Autodesk Fusion 360 part; units mm, degrees
(part 5 of 18)
  spline S23 degree 5 poles (23.1879, -24.3163) (23.1865, -24.3123) (23.1838, -24.3044) (23.1798, -24.2926) (23.1744, -24.2768) (23.1676, -24.2571) (23.1608, -24.2375) (23.154, -24.2179) (23.1471, -24.1984) (23.1403, -24.1789) (23.1334, -24.1595) (23.1265, -24.1401) (23.1197, -24.1208) (23.1128, -24.1016) (23.1058, -24.0823) (23.0989, -24.0632) (23.092, -24.0441) (23.085, -24.025) (23.078, -24.006) (23.071, -23.9871) (23.064, -23.9681) (23.057, -23.9493) (23.05, -23.9305) (23.0429, -23.9118) (23.0359, -23.8931) (23.0288, -23.8744) (23.0217, -23.8558) (23.0147, -23.8373) (23.0076, -23.8188) (23.0004, -23.8004) (22.9933, -23.782) (22.9862, -23.7637) (22.979, -23.7454) (22.9719, -23.7272) (22.9647, -23.7091) (22.9575, -23.691) (22.9503, -23.6729) (22.9431, -23.6549) (22.9359, -23.637) (22.9287, -23.6191) (22.9215, -23.6012) (22.9142, -23.5835) (22.907, -23.5658) (22.8997, -23.5481) (22.8924, -23.5305) (22.8851, -23.5129) (22.8778, -23.4954) (22.8705, -23.478) (22.8632, -23.4606) (22.8559, -23.4433) (22.8486, -23.426) (22.8413, -23.4088) (22.8339, -23.3916) (22.8266, -23.3745) (22.8192, -23.3575) (22.8119, -23.3405) (22.8045, -23.3236) (22.7971, -23.3067) (22.7897, -23.2899) (22.7823, -23.2731) (22.7749, -23.2564) (22.7675, -23.2398) (22.7601, -23.2232) (22.7527, -23.2067) (22.7453, -23.1902) (22.7379, -23.1738) (22.7304, -23.1575) (22.723, -23.1412) (22.7156, -23.125) (22.7081, -23.1088) (22.7007, -23.0927) (22.6932, -23.0766) (22.6858, -23.0607) (22.6783, -23.0447) (22.6709, -23.0289) (22.6634, -23.0131) (22.6559, -22.9973) (22.6485, -22.9816) (22.641, -22.966) (22.6335, -22.9505) (22.626, -22.935) (22.6186, -22.9195) (22.6111, -22.9042) (22.6036, -22.8888) (22.5961, -22.8736) (22.5886, -22.8584) (22.5811, -22.8433) (22.5737, -22.8282) (22.5662, -22.8132) (22.5587, -22.7983) (22.5512, -22.7834) (22.5437, -22.7686) (22.5363, -22.7539) (22.5288, -22.7392) (22.5213, -22.7246) (22.5138, -22.71) (22.5064, -22.6955) (22.4989, -22.6811) (22.4914, -22.6668) (22.484, -22.6525) (22.4765, -22.6383) (22.469, -22.6241) (22.4616, -22.61) (22.4541, -22.596) (22.4467, -22.582) (22.4392, -22.5681) (22.4318, -22.5543) (22.4244, -22.5406) (22.417, -22.5269) (22.4095, -22.5132) (22.4021, -22.4997) (22.3947, -22.4862) (22.3873, -22.4728) (22.3799, -22.4594) (22.3725, -22.4462) (22.3652, -22.4329) (22.3578, -22.4198) (22.3504, -22.4067) (22.3431, -22.3937) (22.3358, -22.3808) (22.3284, -22.3679) (22.3211, -22.3551) (22.3138, -22.3424) (22.3065, -22.3298) (22.2992, -22.3172) (22.2919, -22.3047) (22.2847, -22.2922) (22.2774, -22.2799) (22.2702, -22.2676) (22.2629, -22.2554) (22.2557, -22.2432) (22.2485, -22.2312) (22.2413, -22.2192) (22.2342, -22.2072) (22.227, -22.1954) (22.2199, -22.1836) (22.2127, -22.1719) (22.2056, -22.1603) (22.1985, -22.1487) (22.1915, -22.1372) (22.1844, -22.1258) (22.1774, -22.1145) (22.1703, -22.1033) (22.1633, -22.0921) (22.1564, -22.081) (22.1494, -22.07) (22.1424, -22.059) (22.1355, -22.0482) (22.1286, -22.0374) (22.1217, -22.0267) (22.1149, -22.0161) (22.108, -22.0055) (22.1012, -21.995) (22.0944, -21.9847) (22.0877, -21.9743) (22.0809, -21.9641) (22.0742, -21.954) (22.0675, -21.9439) (22.0609, -21.9339) (22.0542, -21.924) (22.0476, -21.9142) (22.041, -21.9045) (22.0345, -21.8948) (22.028, -21.8853) (22.0215, -21.8758) (22.015, -21.8664) (22.0086, -21.8571) (22.0022, -21.8478) (21.9958, -21.8387) (21.9895, -21.8296) (21.9832, -21.8207) (21.9769, -21.8118) (21.9707, -21.803) (21.9645, -21.7943) (21.9583, -21.7857) (21.9522, -21.7771) (21.9461, -21.7687) (21.9401, -21.7603) (21.9341, -21.7521) (21.9281, -21.7439) (21.9222, -21.7358) (21.9163, -21.7279) (21.9105, -21.72) (21.9047, -21.7122) (21.899, -21.7045) (21.8933, -21.6969) (21.8876, -21.6893) (21.882, -21.6819) (21.8764, -21.6746) (21.8709, -21.6674) (21.8654, -21.6602) (21.86, -21.6532) (21.8547, -21.6463) (21.8494, -21.6394) (21.8441, -21.6327) (21.8389, -21.6261) (21.8338, -21.6195) (21.8287, -21.6131) (21.8237, -21.6068) (21.8187, -21.6005) (21.8138, -21.5944) (21.8089, -21.5884) (21.8042, -21.5825) (21.7994, -21.5767) (21.7948, -21.571) (21.7902, -21.5654) (21.7857, -21.5599) (21.7812, -21.5546) (21.7769, -21.5493) (21.7726, -21.5442) (21.7683, -21.5391) (21.7642, -21.5342) (21.7601, -21.5294) (21.7561, -21.5247) (21.7522, -21.5201) (21.7484, -21.5157) (21.7446, -21.5114) (21.741, -21.5071) (21.7374, -21.5031) (21.7339, -21.4991) (21.7305, -21.4952) (21.7273, -21.4915) (21.7241, -21.4879) (21.721, -21.4845) (21.718, -21.4811) (21.7151, -21.4779) (21.7123, -21.4749) (21.7096, -21.4719) (21.707, -21.4691) (21.7046, -21.4665) (21.7022, -21.464) (21.7, -21.4616) (21.6979, -21.4593) (21.696, -21.4573) (21.6941, -21.4553) (21.6924, -21.4535) (21.6909, -21.4519) (21.6894, -21.4504) (21.6881, -21.4491) (21.687, -21.4479) (21.686, -21.4469) (21.6854, -21.4462) (21.685, -21.4458) (21.6847, -21.4456) (21.6846, -21.4454) knots -1 -1 -1 -1 -1 -1 -0.99583333 -0.99166667 -0.9875 -0.98333333 -0.97916667 -0.975 -0.97083333 -0.96666667 -0.9625 -0.95833333 -0.95416667 -0.95 -0.94583333 -0.94166667 -0.9375 -0.93333333 -0.92916667 -0.925 -0.92083333 -0.91666667 -0.9125 -0.90833333 -0.90416667 -0.9 -0.89583333 -0.89166667 -0.8875 -0.88333333 -0.87916667 -0.875 -0.87083333 -0.86666667 -0.8625 -0.85833333 -0.85416667 -0.85 -0.84583333 -0.84166667 -0.8375 -0.83333333 -0.82916667 -0.825 -0.82083333 -0.81666667 -0.8125 -0.80833333 -0.80416667 -0.8 -0.79583333 -0.79166667 -0.7875 -0.78333333 -0.77916667 -0.775 -0.77083333 -0.76666667 -0.7625 -0.75833333 -0.75416667 -0.75 -0.74583333 -0.74166667 -0.7375 -0.73333333 -0.72916667 -0.725 -0.72083333 -0.71666667 -0.7125 -0.70833333 -0.70416667 -0.7 -0.69583333 -0.69166667 -0.6875 -0.68333333 -0.67916667 -0.675 -0.67083333 -0.66666667 -0.6625 -0.65833333 -0.65416667 -0.65 -0.64583333 -0.64166667 -0.6375 -0.63333333 -0.62916667 -0.625 -0.62083333 -0.61666667 -0.6125 -0.60833333 -0.60416667 -0.6 -0.59583333 -0.59166667 -0.5875 -0.58333333 -0.57916667 -0.575 -0.57083333 -0.56666667 -0.5625 -0.55833333 -0.55416667 -0.55 -0.54583333 -0.54166667 -0.5375 -0.53333333 -0.52916667 -0.525 -0.52083333 -0.51666667 -0.5125 -0.50833333 -0.50416667 -0.5 -0.49583333 -0.49166667 -0.4875 -0.48333333 -0.47916667 -0.475 -0.47083333 -0.46666667 -0.4625 -0.45833333 -0.45416667 -0.45 -0.44583333 -0.44166667 -0.4375 -0.43333333 -0.42916667 -0.425 -0.42083333 -0.41666667 -0.4125 -0.40833333 -0.40416667 -0.4 -0.39583333 -0.39166667 -0.3875 -0.38333333 -0.37916667 -0.375 -0.37083333 -0.36666667 -0.3625 -0.35833333 -0.35416667 -0.35 -0.34583333 -0.34166667 -0.3375 -0.33333333 -0.32916667 -0.325 -0.32083333 -0.31666667 -0.3125 -0.30833333 -0.30416667 -0.3 -0.29583333 -0.29166667 -0.2875 -0.28333333 -0.27916667 -0.275 -0.27083333 -0.26666667 -0.2625 -0.25833333 -0.25416667 -0.25 -0.24583333 -0.24166667 -0.2375 -0.23333333 -0.22916667 -0.225 -0.22083333 -0.21666667 -0.2125 -0.20833333 -0.20416667 -0.2 -0.19583333 -0.19166667 -0.1875 -0.18333333 -0.17916667 -0.175 -0.17083333 -0.16666667 -0.1625 -0.15833333 -0.15416667 -0.15 -0.14583333 -0.14166667 -0.1375 -0.13333333 -0.12916667 -0.125 -0.12083333 -0.11666667 -0.1125 -0.10833333 -0.10416667 -0.1 -0.09583333 -0.09166667 -0.0875 -0.08333333 -0.07916667 -0.075 -0.07083333 -0.06666667 -0.0625 -0.05833333 -0.05416667 -0.05 -0.04583333 -0.04166667 -0.0375 -0.03333333 -0.02916667 -0.025 -0.02083333 -0.01666667 -0.0125 -0.00833333 -0.00416667 0 0 0 0 0 0
  line L46 (21.6846, -21.4454) -> (21.6836, -21.4445)
  line L47 (21.6836, -21.4445) -> (20.5306, -20.3042)
  arc A24 (20.5306, -20.3042) -> (22.339, -18.2958) centre (0, 0) ccw
  line L48 (22.339, -18.2958) -> (23.5936, -19.3233)
  line L49 (23.5936, -19.3233) -> (23.5946, -19.3241)
  spline S24 degree 5 poles (23.5946, -19.3241) (23.5948, -19.3242) (23.595, -19.3245) (23.5955, -19.3248) (23.5962, -19.3254) (23.5973, -19.3263) (23.5986, -19.3273) (23.6001, -19.3284) (23.6017, -19.3297) (23.6035, -19.3311) (23.6054, -19.3326) (23.6076, -19.3342) (23.6098, -19.336) (23.6123, -19.3378) (23.6149, -19.3398) (23.6176, -19.3418) (23.6205, -19.344) (23.6236, -19.3462) (23.6268, -19.3486) (23.6301, -19.3511) (23.6336, -19.3536) (23.6372, -19.3562) (23.641, -19.3589) (23.6449, -19.3618) (23.649, -19.3646) (23.6531, -19.3676) (23.6574, -19.3707) (23.6619, -19.3738) (23.6665, -19.377) (23.6712, -19.3802) (23.676, -19.3836) (23.6809, -19.387) (23.686, -19.3905) (23.6912, -19.394) (23.6965, -19.3976) (23.702, -19.4013) (23.7076, -19.4051) (23.7132, -19.4089) (23.7191, -19.4127) (23.725, -19.4166) (23.731, -19.4206) (23.7372, -19.4246) (23.7434, -19.4287) (23.7498, -19.4329) (23.7563, -19.4371) (23.7629, -19.4413) (23.7696, -19.4456) (23.7764, -19.4499) (23.7834, -19.4543) (23.7904, -19.4587) (23.7975, -19.4632) (23.8048, -19.4677) (23.8121, -19.4723) (23.8196, -19.4769) (23.8271, -19.4816) (23.8348, -19.4862) (23.8426, -19.491) (23.8504, -19.4957) (23.8584, -19.5005) (23.8665, -19.5054) (23.8746, -19.5103) (23.8829, -19.5152) (23.8913, -19.5201) (23.8997, -19.5251) (23.9083, -19.5301) (23.9169, -19.5352) (23.9257, -19.5402) (23.9345, -19.5453) (23.9434, -19.5505) (23.9525, -19.5556) (23.9616, -19.5608) (23.9708, -19.5661) (23.9801, -19.5713) (23.9895, -19.5766) (23.999, -19.5819) (24.0086, -19.5872) (24.0182, -19.5926) (24.028, -19.5979) (24.0379, -19.6033) (24.0478, -19.6088) (24.0578, -19.6142) (24.0679, -19.6197) (24.0781, -19.6252) (24.0884, -19.6307) (24.0988, -19.6362) (24.1092, -19.6417) (24.1198, -19.6473) (24.1304, -19.6529) (24.1411, -19.6585) (24.1519, -19.6641) (24.1628, -19.6697) (24.1737, -19.6754) (24.1848, -19.6811) (24.1959, -19.6867) (24.2071, -19.6924) (24.2184, -19.6981) (24.2297, -19.7039) (24.2412, -19.7096) (24.2527, -19.7154) (24.2643, -19.7211) (24.276, -19.7269) (24.2878, -19.7327) (24.2996, -19.7385) (24.3115, -19.7443) (24.3235, -19.7501) (24.3356, -19.7559) (24.3478, -19.7618) (24.36, -19.7676) (24.3723, -19.7735) (24.3847, -19.7793) (24.3971, -19.7852) (24.4097, -19.7911) (24.4223, -19.797) (24.435, -19.8029) (24.4477, -19.8088) (24.4606, -19.8147) (24.4735, -19.8206) (24.4865, -19.8265) (24.4995, -19.8324) (24.5126, -19.8383) (24.5258, -19.8443) (24.5391, -19.8502) (24.5525, -19.8561) (24.5659, -19.8621) (24.5794, -19.868) (24.5929, -19.874) (24.6065, -19.8799) (24.6202, -19.8859) (24.634, -19.8918) (24.6479, -19.8978) (24.6618, -19.9037) (24.6757, -19.9097) (24.6898, -19.9156) (24.7039, -19.9216) (24.7181, -19.9275) (24.7324, -19.9335) (24.7467, -19.9395) (24.7611, -19.9454) (24.7755, -19.9514) (24.7901, -19.9573) (24.8046, -19.9633) (24.8193, -19.9692) (24.834, -19.9751) (24.8488, -19.9811) (24.8637, -19.987) (24.8786, -19.993) (24.8936, -19.9989) (24.9087, -20.0048) (24.9238, -20.0107) (24.939, -20.0166) (24.9542, -20.0226) (24.9695, -20.0285) (24.9849, -20.0344) (25.0004, -20.0403) (25.0159, -20.0462) (25.0314, -20.052) (25.0471, -20.0579) (25.0628, -20.0638) (25.0785, -20.0697) (25.0943, -20.0755) (25.1102, -20.0814) (25.1262, -20.0872) (25.1422, -20.0931) (25.1583, -20.0989) (25.1744, -20.1047) (25.1906, -20.1105) (25.2068, -20.1164) (25.2232, -20.1222) (25.2395, -20.1279) (25.256, -20.1337) (25.2725, -20.1395) (25.289, -20.1453) (25.3056, -20.151) (25.3223, -20.1568) (25.3391, -20.1625) (25.3559, -20.1682) (25.3727, -20.1739) (25.3896, -20.1796) (25.4066, -20.1853) (25.4236, -20.191) (25.4407, -20.1967) (25.4579, -20.2023) (25.4751, -20.208) (25.4923, -20.2136) (25.5097, -20.2192) (25.527, -20.2248) (25.5445, -20.2304) (25.562, -20.236) (25.5795, -20.2416) (25.5971, -20.2471) (25.6148, -20.2527) (25.6325, -20.2582) (25.6503, -20.2637) (25.6681, -20.2693) (25.686, -20.2747) (25.7039, -20.2802) (25.7219, -20.2857) (25.74, -20.2911) (25.7581, -20.2966) (25.7763, -20.302) (25.7945, -20.3074) (25.8128, -20.3128) (25.8311, -20.3182) (25.8495, -20.3235) (25.8679, -20.3289) (25.8864, -20.3342) (25.9049, -20.3395) (25.9235, -20.3448) (25.9422, -20.3501) (25.9609, -20.3554) (25.9796, -20.3606) (25.9984, -20.3659) (26.0173, -20.3711) (26.0362, -20.3763) (26.0552, -20.3815) (26.0742, -20.3866) (26.0933, -20.3918) (26.1124, -20.3969) (26.1316, -20.402) (26.1508, -20.4071) (26.1701, -20.4122) (26.1894, -20.4173) (26.2088, -20.4223) (26.2282, -20.4273) (26.2477, -20.4323) (26.2672, -20.4373) (26.2868, -20.4423) (26.3064, -20.4472) (26.3261, -20.4522) (26.3459, -20.4571) (26.3656, -20.462) (26.3855, -20.4668) (26.4054, -20.4717) (26.4253, -20.4765) (26.4453, -20.4813) (26.4653, -20.4861) (26.4854, -20.4909) (26.5055, -20.4957) (26.5257, -20.5004) (26.5459, -20.5051) (26.5662, -20.5098) (26.5824, -20.5135) (26.5946, -20.5163) (26.6028, -20.5182) (26.6069, -20.5191) knots 0 0 0 0 0 0 0.00416667 0.00833333 0.0125 0.01666667 0.02083333 0.025 0.02916667 0.03333333 0.0375 0.04166667 0.04583333 0.05 0.05416667 0.05833333 0.0625 0.06666667 0.07083333 0.075 0.07916667 0.08333333 0.0875 0.09166667 0.09583333 0.1 0.10416667 0.10833333 0.1125 0.11666667 0.12083333 0.125 0.12916667 0.13333333 0.1375 0.14166667 0.14583333 0.15 0.15416667 0.15833333 0.1625 0.16666667 0.17083333 0.175 0.17916667 0.18333333 0.1875 0.19166667 0.19583333 0.2 0.20416667 0.20833333 0.2125 0.21666667 0.22083333 0.225 0.22916667 0.23333333 0.2375 0.24166667 0.24583333 0.25 0.25416667 0.25833333 0.2625 0.26666667 0.27083333 0.275 0.27916667 0.28333333 0.2875 0.29166667 0.29583333 0.3 0.30416667 0.30833333 0.3125 0.31666667 0.32083333 0.325 0.32916667 0.33333333 0.3375 0.34166667 0.34583333 0.35 0.35416667 0.35833333 0.3625 0.36666667 0.37083333 0.375 0.37916667 0.38333333 0.3875 0.39166667 0.39583333 0.4 0.40416667 0.40833333 0.4125 0.41666667 0.42083333 0.425 0.42916667 0.43333333 0.4375 0.44166667 0.44583333 0.45 0.45416667 0.45833333 0.4625 0.46666667 0.47083333 0.475 0.47916667 0.48333333 0.4875 0.49166667 0.49583333 0.5 0.50416667 0.50833333 0.5125 0.51666667 0.52083333 0.525 0.52916667 0.53333333 0.5375 0.54166667 0.54583333 0.55 0.55416667 0.55833333 0.5625 0.56666667 0.57083333 0.575 0.57916667 0.58333333 0.5875 0.59166667 0.59583333 0.6 0.60416667 0.60833333 0.6125 0.61666667 0.62083333 0.625 0.62916667 0.63333333 0.6375 0.64166667 0.64583333 0.65 0.65416667 0.65833333 0.6625 0.66666667 0.67083333 0.675 0.67916667 0.68333333 0.6875 0.69166667 0.69583333 0.7 0.70416667 0.70833333 0.7125 0.71666667 0.72083333 0.725 0.72916667 0.73333333 0.7375 0.74166667 0.74583333 0.75 0.75416667 0.75833333 0.7625 0.76666667 0.77083333 0.775 0.77916667 0.78333333 0.7875 0.79166667 0.79583333 0.8 0.80416667 0.80833333 0.8125 0.81666667 0.82083333 0.825 0.82916667 0.83333333 0.8375 0.84166667 0.84583333 0.85 0.85416667 0.85833333 0.8625 0.86666667 0.87083333 0.875 0.87916667 0.88333333 0.8875 0.89166667 0.89583333 0.9 0.90416667 0.90833333 0.9125 0.91666667 0.92083333 0.925 0.92916667 0.93333333 0.9375 0.94166667 0.94583333 0.95 0.95416667 0.95833333 0.9625 0.96666667 0.97083333 0.975 0.97916667 0.98333333 0.9875 0.99166667 0.99583333 1 1 1 1 1 1
  arc A25 (26.6069, -20.5191) -> (27.7368, -18.9639) centre (0, 0) ccw
  spline S25 degree 5 poles (27.7368, -18.9639) (27.7347, -18.9603) (27.7304, -18.9531) (27.724, -18.9424) (27.7154, -18.9281) (27.7046, -18.9102) (27.6939, -18.8924) (27.6832, -18.8747) (27.6724, -18.857) (27.6617, -18.8394) (27.6509, -18.8219) (27.6402, -18.8043) (27.6294, -18.7869) (27.6187, -18.7695) (27.6079, -18.7521) (27.5972, -18.7348) (27.5864, -18.7176) (27.5756, -18.7004) (27.5648, -18.6832) (27.5541, -18.6661) (27.5433, -18.6491) (27.5325, -18.6321) (27.5217, -18.6152) (27.5109, -18.5983) (27.5001, -18.5815) (27.4894, -18.5647) (27.4786, -18.548) (27.4678, -18.5314) (27.457, -18.5148) (27.4462, -18.4982) (27.4354, -18.4817) (27.4246, -18.4653) (27.4138, -18.4489) (27.403, -18.4326) (27.3923, -18.4163) (27.3815, -18.4001) (27.3707, -18.3839) (27.3599, -18.3678) (27.3491, -18.3518) (27.3383, -18.3358) (27.3275, -18.3199) (27.3168, -18.304) (27.306, -18.2882) (27.2952, -18.2724) (27.2844, -18.2567) (27.2737, -18.241) (27.2629, -18.2254) (27.2521, -18.2099) (27.2414, -18.1944) (27.2306, -18.179) (27.2198, -18.1636) (27.2091, -18.1483) (27.1983, -18.133) (27.1876, -18.1178) (27.1769, -18.1027) (27.1661, -18.0876) (27.1554, -18.0726) (27.1447, -18.0576) (27.134, -18.0427) (27.1232, -18.0278) (27.1125, -18.013) (27.1018, -17.9983) (27.0911, -17.9836) (27.0805, -17.969) (27.0698, -17.9545) (27.0591, -17.9399) (27.0484, -17.9255) (27.0378, -17.9111) (27.0271, -17.8968) (27.0165, -17.8825) (27.0059, -17.8683) (26.9952, -17.8542) (26.9846, -17.8401) (26.974, -17.8261) (26.9634, -17.8121) (26.9528, -17.7982) (26.9423, -17.7843) (26.9317, -17.7706) (26.9211, -17.7568) (26.9106, -17.7432) (26.9, -17.7296) (26.8895, -17.716) (26.879, -17.7025) (26.8685, -17.6891) (26.858, -17.6758) (26.8475, -17.6625) (26.8371, -17.6492) (26.8266, -17.636) (26.8162, -17.6229) (26.8058, -17.6099) (26.7954, -17.5969) (26.785, -17.584) (26.7746, -17.5711) (26.7642, -17.5583) (26.7539, -17.5456) (26.7435, -17.5329) (26.7332, -17.5203) (26.7229, -17.5077) (26.7126, -17.4952) (26.7023, -17.4828) (26.6921, -17.4704) (26.6818, -17.4581) (26.6716, -17.4459) (26.6614, -17.4337) (26.6512, -17.4216) (26.6411, -17.4096) (26.6309, -17.3976) (26.6208, -17.3857) (26.6107, -17.3739) (26.6006, -17.3621) (26.5905, -17.3504) (26.5805, -17.3387) (26.5705, -17.3271) (26.5605, -17.3156) (26.5505, -17.3041) (26.5405, -17.2928) (26.5306, -17.2814) (26.5207, -17.2702) (26.5108, -17.259) (26.5009, -17.2479) (26.4911, -17.2368) (26.4812, -17.2258) (26.4714, -17.2149) (26.4617, -17.204) (26.4519, -17.1932) (26.4422, -17.1825) (26.4325, -17.1719) (26.4228, -17.1613) (26.4132, -17.1508) (26.4036, -17.1403) (26.394, -17.1299) (26.3845, -17.1196) (26.3749, -17.1094) (26.3654, -17.0992) (26.356, -17.0891) (26.3465, -17.0791) (26.3371, -17.0691) (26.3278, -17.0592) (26.3184, -17.0494) (26.3091, -17.0396) (26.2998, -17.0299) (26.2906, -17.0203) (26.2814, -17.0108) (26.2722, -17.0013) (26.2631, -16.9919) (26.254, -16.9826) (26.2449, -16.9733) (26.2359, -16.9641) (26.2269, -16.955) (26.2179, -16.946) (26.209, -16.937) (26.2001, -16.9281) (26.1913, -16.9193) (26.1825, -16.9105) (26.1737, -16.9019) (26.165, -16.8933) (26.1563, -16.8847) (26.1477, -16.8763) (26.1391, -16.8679) (26.1306, -16.8596) (26.1221, -16.8514) (26.1136, -16.8432) (26.1052, -16.8351) (26.0968, -16.8271) (26.0885, -16.8192) (26.0802, -16.8114) (26.072, -16.8036) (26.0638, -16.7959) (26.0557, -16.7883) (26.0476, -16.7807) (26.0396, -16.7733) (26.0316, -16.7659) (26.0237, -16.7586) (26.0158, -16.7513) (26.008, -16.7442) (26.0002, -16.7371) (25.9925, -16.7301) (25.9849, -16.7232) (25.9773, -16.7164) (25.9698, -16.7096) (25.9623, -16.703) (25.9549, -16.6964) (25.9475, -16.6899) (25.9402, -16.6835) (25.933, -16.6771) (25.9259, -16.6709) (25.9188, -16.6647) (25.9117, -16.6586) (25.9048, -16.6526) (25.8979, -16.6467) (25.891, -16.6408) (25.8843, -16.6351) (25.8776, -16.6294) (25.871, -16.6238) (25.8645, -16.6183) (25.858, -16.6129) (25.8516, -16.6076) (25.8453, -16.6024) (25.8391, -16.5972) (25.8329, -16.5922) (25.8268, -16.5872) (25.8208, -16.5823) (25.8149, -16.5775) (25.8091, -16.5728) (25.8034, -16.5682) (25.7977, -16.5637) (25.7922, -16.5593) (25.7867, -16.555) (25.7813, -16.5507) (25.7761, -16.5466) (25.7709, -16.5426) (25.7658, -16.5386) (25.7608, -16.5348) (25.7559, -16.531) (25.7512, -16.5273) (25.7465, -16.5238) (25.7419, -16.5203) (25.7375, -16.517) (25.7331, -16.5137) (25.7289, -16.5105) (25.7248, -16.5075) (25.7208, -16.5045) (25.7169, -16.5017) (25.7132, -16.4989) (25.7096, -16.4963) (25.7061, -16.4938) (25.7027, -16.4914) (25.6995, -16.489) (25.6964, -16.4868) (25.6934, -16.4847) (25.6906, -16.4828) (25.6879, -16.4809) (25.6854, -16.4792) (25.6831, -16.4775) (25.6809, -16.476) (25.6788, -16.4746) (25.677, -16.4733) (25.6753, -16.4722) (25.6737, -16.4711) (25.6724, -16.4702) (25.6712, -16.4695) (25.6704, -16.4689) (25.6699, -16.4686) (25.6696, -16.4684) (25.6695, -16.4683) knots -1 -1 -1 -1 -1 -1 -0.99583333 -0.99166667 -0.9875 -0.98333333 -0.97916667 -0.975 -0.97083333 -0.96666667 -0.9625 -0.95833333 -0.95416667 -0.95 -0.94583333 -0.94166667 -0.9375 -0.93333333 -0.92916667 -0.925 -0.92083333 -0.91666667 -0.9125 -0.90833333 -0.90416667 -0.9 -0.89583333 -0.89166667 -0.8875 -0.88333333 -0.87916667 -0.875 -0.87083333 -0.86666667 -0.8625 -0.85833333 -0.85416667 -0.85 -0.84583333 -0.84166667 -0.8375 -0.83333333 -0.82916667 -0.825 -0.82083333 -0.81666667 -0.8125 -0.80833333 -0.80416667 -0.8 -0.79583333 -0.79166667 -0.7875 -0.78333333 -0.77916667 -0.775 -0.77083333 -0.76666667 -0.7625 -0.75833333 -0.75416667 -0.75 -0.74583333 -0.74166667 -0.7375 -0.73333333 -0.72916667 -0.725 -0.72083333 -0.71666667 -0.7125 -0.70833333 -0.70416667 -0.7 -0.69583333 -0.69166667 -0.6875 -0.68333333 -0.67916667 -0.675 -0.67083333 -0.66666667 -0.6625 -0.65833333 -0.65416667 -0.65 -0.64583333 -0.64166667 -0.6375 -0.63333333 -0.62916667 -0.625 -0.62083333 -0.61666667 -0.6125 -0.60833333 -0.60416667 -0.6 -0.59583333 -0.59166667 -0.5875 -0.58333333 -0.57916667 -0.575 -0.57083333 -0.56666667 -0.5625 -0.55833333 -0.55416667 -0.55 -0.54583333 -0.54166667 -0.5375 -0.53333333 -0.52916667 -0.525 -0.52083333 -0.51666667 -0.5125 -0.50833333 -0.50416667 -0.5 -0.49583333 -0.49166667 -0.4875 -0.48333333 -0.47916667 -0.475 -0.47083333 -0.46666667 -0.4625 -0.45833333 -0.45416667 -0.45 -0.44583333 -0.44166667 -0.4375 -0.43333333 -0.42916667 -0.425 -0.42083333 -0.41666667 -0.4125 -0.40833333 -0.40416667 -0.4 -0.39583333 -0.39166667 -0.3875 -0.38333333 -0.37916667 -0.375 -0.37083333 -0.36666667 -0.3625 -0.35833333 -0.35416667 -0.35 -0.34583333 -0.34166667 -0.3375 -0.33333333 -0.32916667 -0.325 -0.32083333 -0.31666667 -0.3125 -0.30833333 -0.30416667 -0.3 -0.29583333 -0.29166667 -0.2875 -0.28333333 -0.27916667 -0.275 -0.27083333 -0.26666667 -0.2625 -0.25833333 -0.25416667 -0.25 -0.24583333 -0.24166667 -0.2375 -0.23333333 -0.22916667 -0.225 -0.22083333 -0.21666667 -0.2125 -0.20833333 -0.20416667 -0.2 -0.19583333 -0.19166667 -0.1875 -0.18333333 -0.17916667 -0.175 -0.17083333 -0.16666667 -0.1625 -0.15833333 -0.15416667 -0.15 -0.14583333 -0.14166667 -0.1375 -0.13333333 -0.12916667 -0.125 -0.12083333 -0.11666667 -0.1125 -0.10833333 -0.10416667 -0.1 -0.09583333 -0.09166667 -0.0875 -0.08333333 -0.07916667 -0.075 -0.07083333 -0.06666667 -0.0625 -0.05833333 -0.05416667 -0.05 -0.04583333 -0.04166667 -0.0375 -0.03333333 -0.02916667 -0.025 -0.02083333 -0.01666667 -0.0125 -0.00833333 -0.00416667 0 0 0 0 0 0
  line L50 (25.6695, -16.4683) -> (25.6683, -16.4676)
  line L51 (25.6683, -16.4676) -> (24.3034, -15.5919)
  arc A26 (24.3034, -15.5919) -> (25.6547, -13.2514) centre (0, 0) ccw
  line L52 (25.6547, -13.2514) -> (27.0955, -13.9956)
  line L53 (27.0955, -13.9956) -> (27.0967, -13.9963)
  spline S26 degree 5 poles (27.0967, -13.9963) (27.0969, -13.9963) (27.0972, -13.9965) (27.0977, -13.9968) (27.0986, -13.9972) (27.0998, -13.9978) (27.1013, -13.9985) (27.1029, -13.9993) (27.1048, -14.0002) (27.1068, -14.0012) (27.1091, -14.0023) (27.1115, -14.0034) (27.1141, -14.0047) (27.1169, -14.006) (27.1198, -14.0073) (27.1229, -14.0088) (27.1262, -14.0103) (27.1297, -14.0119) (27.1333, -14.0135) (27.1371, -14.0152) (27.141, -14.017) (27.1451, -14.0188) (27.1493, -14.0207) (27.1537, -14.0226) (27.1583, -14.0246) (27.163, -14.0266) (27.1679, -14.0287) (27.1728, -14.0308) (27.178, -14.033) (27.1833, -14.0352) (27.1887, -14.0375) (27.1942, -14.0398) (27.1999, -14.0422) (27.2058, -14.0445) (27.2117, -14.047) (27.2178, -14.0494) (27.224, -14.0519) (27.2304, -14.0545) (27.2369, -14.057) (27.2435, -14.0596) (27.2502, -14.0623) (27.2571, -14.0649) (27.264, -14.0676) (27.2711, -14.0703) (27.2784, -14.0731) (27.2857, -14.0759) (27.2931, -14.0787) (27.3007, -14.0815) (27.3084, -14.0843) (27.3162, -14.0872) (27.3241, -14.0901) (27.3322, -14.093) (27.3403, -14.096) (27.3485, -14.0989) (27.3569, -14.1019) (27.3654, -14.1049) (27.374, -14.1079) (27.3826, -14.1109) (27.3914, -14.114) (27.4003, -14.117) (27.4093, -14.1201) (27.4184, -14.1232) (27.4276, -14.1263) (27.4369, -14.1294) (27.4464, -14.1325) (27.4559, -14.1357) (27.4655, -14.1388) (27.4752, -14.142) (27.485, -14.1451) (27.4949, -14.1483) (27.5049, -14.1515) (27.515, -14.1547) (27.5252, -14.1579) (27.5355, -14.1611) (27.5459, -14.1643) (27.5563, -14.1675) (27.5669, -14.1707) (27.5776, -14.174) (27.5883, -14.1772) (27.5992, -14.1804) (27.6101, -14.1837) (27.6211, -14.1869) (27.6323, -14.1902) (27.6435, -14.1934) (27.6547, -14.1967) (27.6661, -14.1999) (27.6776, -14.2032) (27.6891, -14.2064) (27.7008, -14.2097) (27.7125, -14.2129) (27.7243, -14.2162) (27.7362, -14.2194) (27.7482, -14.2227) (27.7602, -14.2259) (27.7724, -14.2292) (27.7846, -14.2324) (27.7969, -14.2356) (27.8093, -14.2389) (27.8218, -14.2421) (27.8343, -14.2453) (27.847, -14.2485) (27.8597, -14.2518) (27.8725, -14.255) (27.8853, -14.2582) (27.8983, -14.2614) (27.9113, -14.2646) (27.9244, -14.2677) (27.9376, -14.2709) (27.9508, -14.2741) (27.9642, -14.2772) (27.9776, -14.2804) (27.9911, -14.2835) (28.0046, -14.2867) (28.0183, -14.2898) (28.032, -14.2929) (28.0457, -14.296) (28.0596, -14.2991) (28.0735, -14.3022) (28.0875, -14.3053) (28.1016, -14.3084) (28.1157, -14.3114) (28.13, -14.3145) (28.1442, -14.3175) (28.1586, -14.3205) (28.173, -14.3235) (28.1875, -14.3265) (28.2021, -14.3295) (28.2167, -14.3325) (28.2314, -14.3354) (28.2462, -14.3384) (28.2611, -14.3413) (28.276, -14.3442) (28.291, -14.3471) (28.306, -14.35) (28.3211, -14.3529) (28.3363, -14.3558) (28.3515, -14.3586) (28.3669, -14.3614) (28.3822, -14.3643) (28.3977, -14.367) (28.4132, -14.3698) (28.4288, -14.3726) (28.4444, -14.3754) (28.4601, -14.3781) (28.4759, -14.3808) (28.4917, -14.3835) (28.5076, -14.3862) (28.5236, -14.3889) (28.5396, -14.3915) (28.5557, -14.3941) (28.5718, -14.3967) (28.588, -14.3993) (28.6043, -14.4019) (28.6206, -14.4045) (28.637, -14.407) (28.6535, -14.4095) (28.67, -14.412) (28.6866, -14.4145) (28.7032, -14.417) (28.7199, -14.4194) (28.7367, -14.4219) (28.7535, -14.4243) (28.7704, -14.4266) (28.7873, -14.429) (28.8043, -14.4313) (28.8213, -14.4337) (28.8384, -14.436) (28.8556, -14.4382) (28.8728, -14.4405) (28.8901, -14.4427) (28.9074, -14.445) (28.9248, -14.4471) (28.9423, -14.4493) (28.9598, -14.4515) (28.9774, -14.4536) (28.995, -14.4557) (29.0126, -14.4578) (29.0304, -14.4598) (29.0482, -14.4619) (29.066, -14.4639) (29.0839, -14.4659) (29.1019, -14.4679) (29.1199, -14.4698) (29.1379, -14.4717) (29.156, -14.4736) (29.1742, -14.4755) (29.1924, -14.4774) (29.2107, -14.4792) (29.229, -14.481) (29.2474, -14.4828) (29.2658, -14.4845) (29.2843, -14.4862) (29.3028, -14.4879) (29.3214, -14.4896) (29.3401, -14.4913) (29.3587, -14.4929) (29.3775, -14.4945) (29.3963, -14.4961) (29.4151, -14.4976) (29.434, -14.4992) (29.453, -14.5007) (29.472, -14.5021) (29.491, -14.5036) (29.5101, -14.505) (29.5292, -14.5064) (29.5484, -14.5078) (29.5677, -14.5091) (29.587, -14.5104) (29.6063, -14.5117) (29.6257, -14.513) (29.6451, -14.5142) (29.6646, -14.5154) (29.6842, -14.5166) (29.7037, -14.5178) (29.7234, -14.5189) (29.743, -14.52) (29.7628, -14.5211) (29.7825, -14.5221) (29.8024, -14.5231) (29.8222, -14.5241) (29.8421, -14.5251) (29.8621, -14.526) (29.8821, -14.5269) (29.9021, -14.5278) (29.9222, -14.5286) (29.9424, -14.5294) (29.9626, -14.5302) (29.9828, -14.531) (30.0031, -14.5317) (30.0234, -14.5324) (30.0438, -14.5331) (30.0642, -14.5337) (30.0846, -14.5344) (30.1051, -14.5349) (30.1257, -14.5355) (30.1463, -14.536) (30.1669, -14.5365) (30.1876, -14.537) (30.2083, -14.5374) (30.2291, -14.5378) (30.2499, -14.5382) (30.2665, -14.5385) (30.2791, -14.5387) (30.2874, -14.5388) (30.2916, -14.5388) knots 0 0 0 0 0 0 0.00416667 0.00833333 0.0125 0.01666667 0.02083333 0.025 0.02916667 0.03333333 0.0375 0.04166667 0.04583333 0.05 0.05416667 0.05833333 0.0625 0.06666667 0.07083333 0.075 0.07916667 0.08333333 0.0875 0.09166667 0.09583333 0.1 0.10416667 0.10833333 0.1125 0.11666667 0.12083333 0.125 0.12916667 0.13333333 0.1375 0.14166667 0.14583333 0.15 0.15416667 0.15833333 0.1625 0.16666667 0.17083333 0.175 0.17916667 0.18333333 0.1875 0.19166667 0.19583333 0.2 0.20416667 0.20833333 0.2125 0.21666667 0.22083333 0.225 0.22916667 0.23333333 0.2375 0.24166667 0.24583333 0.25 0.25416667 0.25833333 0.2625 0.26666667 0.27083333 0.275 0.27916667 0.28333333 0.2875 0.29166667 0.29583333 0.3 0.30416667 0.30833333 0.3125 0.31666667 0.32083333 0.325 0.32916667 0.33333333 0.3375 0.34166667 0.34583333 0.35 0.35416667 0.35833333 0.3625 0.36666667 0.37083333 0.375 0.37916667 0.38333333 0.3875 0.39166667 0.39583333 0.4 0.40416667 0.40833333 0.4125 0.41666667 0.42083333 0.425 0.42916667 0.43333333 0.4375 0.44166667 0.44583333 0.45 0.45416667 0.45833333 0.4625 0.46666667 0.47083333 0.475 0.47916667 0.48333333 0.4875 0.49166667 0.49583333 0.5 0.50416667 0.50833333 0.5125 0.51666667 0.52083333 0.525 0.52916667 0.53333333 0.5375 0.54166667 0.54583333 0.55 0.55416667 0.55833333 0.5625 0.56666667 0.57083333 0.575 0.57916667 0.58333333 0.5875 0.59166667 0.59583333 0.6 0.60416667 0.60833333 0.6125 0.61666667 0.62083333 0.625 0.62916667 0.63333333 0.6375 0.64166667 0.64583333 0.65 0.65416667 0.65833333 0.6625 0.66666667 0.67083333 0.675 0.67916667 0.68333333 0.6875 0.69166667 0.69583333 0.7 0.70416667 0.70833333 0.7125 0.71666667 0.72083333 0.725 0.72916667 0.73333333 0.7375 0.74166667 0.74583333 0.75 0.75416667 0.75833333 0.7625 0.76666667 0.77083333 0.775 0.77916667 0.78333333 0.7875 0.79166667 0.79583333 0.8 0.80416667 0.80833333 0.8125 0.81666667 0.82083333 0.825 0.82916667 0.83333333 0.8375 0.84166667 0.84583333 0.85 0.85416667 0.85833333 0.8625 0.86666667 0.87083333 0.875 0.87916667 0.88333333 0.8875 0.89166667 0.89583333 0.9 0.90416667 0.90833333 0.9125 0.91666667 0.92083333 0.925 0.92916667 0.93333333 0.9375 0.94166667 0.94583333 0.95 0.95416667 0.95833333 0.9625 0.96666667 0.97083333 0.975 0.97916667 0.98333333 0.9875 0.99166667 0.99583333 1 1 1 1 1 1
  arc A27 (30.2916, -14.5388) -> (31.0735, -12.7827) centre (0, 0) ccw
  spline S27 degree 5 poles (31.0735, -12.7827) (31.0707, -12.7796) (31.065, -12.7735) (31.0565, -12.7643) (31.0451, -12.7521) (31.0309, -12.7369) (31.0167, -12.7217) (31.0025, -12.7066) (30.9883, -12.6916) (30.9742, -12.6765) (30.96, -12.6616) (30.9458, -12.6467) (30.9317, -12.6319) (30.9175, -12.6171) (30.9034, -12.6023) (30.8893, -12.5876) (30.8752, -12.573) (30.861, -12.5584) (30.8469, -12.5439) (30.8328, -12.5294) (30.8188, -12.515) (30.8047, -12.5006) (30.7906, -12.4863) (30.7766, -12.4721) (30.7625, -12.4579) (30.7485, -12.4437) (30.7345, -12.4296) (30.7204, -12.4155) (30.7064, -12.4016) (30.6924, -12.3876) (30.6785, -12.3737) (30.6645, -12.3599) (30.6505, -12.3461) (30.6366, -12.3324) (30.6226, -12.3187) (30.6087, -12.3051) (30.5948, -12.2915) (30.5809, -12.278) (30.567, -12.2646) (30.5531, -12.2512) (30.5393, -12.2378) (30.5254, -12.2245) (30.5116, -12.2113) (30.4978, -12.1981) (30.484, -12.185) (30.4702, -12.1719) (30.4564, -12.1589) (30.4426, -12.1459) (30.4289, -12.133) (30.4152, -12.1202) (30.4014, -12.1074) (30.3877, -12.0946) (30.3741, -12.0819) (30.3604, -12.0693) (30.3467, -12.0567) (30.3331, -12.0442) (30.3195, -12.0317) (30.3059, -12.0193) (30.2923, -12.0069) (30.2787, -11.9946) (30.2652, -11.9824) (30.2517, -11.9702) (30.2382, -11.9581) (30.2247, -11.946) (30.2112, -11.934) (30.1977, -11.922) (30.1843, -11.9101) (30.1709, -11.8982) (30.1575, -11.8865) (30.1441, -11.8747) (30.1308, -11.863) (30.1174, -11.8514) (30.1041, -11.8398) (30.0908, -11.8283) (30.0775, -11.8169) (30.0643, -11.8055) (30.0511, -11.7941) (30.0379, -11.7828) (30.0247, -11.7716) (30.0115, -11.7604) (29.9984, -11.7493) (29.9853, -11.7382) (29.9722, -11.7272) (29.9591, -11.7163) (29.9461, -11.7054) (29.9331, -11.6946) (29.9201, -11.6838) (29.9071, -11.6731) (29.8942, -11.6624) (29.8813, -11.6518) (29.8684, -11.6413) (29.8556, -11.6308) (29.8427, -11.6204) (29.8299, -11.61) (29.8172, -11.5997) (29.8044, -11.5895) (29.7917, -11.5793) (29.779, -11.5691) (29.7663, -11.559) (29.7537, -11.549) (29.7411, -11.5391) (29.7285, -11.5292) (29.716, -11.5193) (29.7035, -11.5095) (29.691, -11.4998) (29.6786, -11.4902) (29.6661, -11.4806) (29.6538, -11.471) (29.6414, -11.4615) (29.6291, -11.4521) (29.6168, -11.4427) (29.6046, -11.4334) (29.5923, -11.4242) (29.5802, -11.415) (29.568, -11.4059) (29.5559, -11.3968) (29.5438, -11.3878) (29.5318, -11.3788) (29.5198, -11.3699) (29.5078, -11.3611) (29.4959, -11.3523) (29.484, -11.3436) (29.4721, -11.335) (29.4603, -11.3264) (29.4486, -11.3179) (29.4368, -11.3094) (29.4251, -11.301) (29.4135, -11.2926) (29.4019, -11.2844) (29.3903, -11.2761) (29.3788, -11.268) (29.3673, -11.2599) (29.3558, -11.2518) (29.3444, -11.2439) (29.3331, -11.2359) (29.3217, -11.2281) (29.3105, -11.2203) (29.2993, -11.2126) (29.2881, -11.2049) (29.2769, -11.1973) (29.2659, -11.1897) (29.2548, -11.1823) (29.2438, -11.1748) (29.2329, -11.1675) (29.222, -11.1602) (29.2111, -11.153) (29.2004, -11.1458) (29.1896, -11.1387) (29.1789, -11.1316) (29.1683, -11.1247) (29.1577, -11.1177) (29.1472, -11.1109) (29.1367, -11.1041) (29.1262, -11.0974) (29.1159, -11.0907) (29.1056, -11.0841) (29.0953, -11.0776) (29.0851, -11.0711) (29.0749, -11.0647) (29.0649, -11.0583) (29.0548, -11.052) (29.0449, -11.0458) (29.0349, -11.0397) (29.0251, -11.0336) (29.0153, -11.0276) (29.0056, -11.0216) (28.9959, -11.0157) (28.9863, -11.0099) (28.9768, -11.0041) (28.9673, -10.9984) (28.9579, -10.9928) (28.9486, -10.9872) (28.9393, -10.9817) (28.9301, -10.9763) (28.921, -10.9709) (28.9119, -10.9656) (28.9029, -10.9604) (28.894, -10.9552) (28.8852, -10.9501) (28.8764, -10.9451) (28.8677, -10.9401) (28.8591, -10.9352) (28.8505, -10.9304) (28.8421, -10.9256) (28.8337, -10.9209) (28.8254, -10.9163) (28.8172, -10.9117) (28.809, -10.9072) (28.801, -10.9028) (28.793, -10.8984) (28.7851, -10.8941) (28.7773, -10.8899) (28.7696, -10.8858) (28.7619, -10.8817) (28.7544, -10.8777) (28.747, -10.8737) (28.7396, -10.8698) (28.7323, -10.866) (28.7252, -10.8623) (28.7181, -10.8586) (28.7111, -10.855) (28.7043, -10.8515) (28.6975, -10.848) (28.6908, -10.8447) (28.6842, -10.8414) (28.6778, -10.8381) (28.6714, -10.8349) (28.6652, -10.8318) (28.6591, -10.8288) (28.653, -10.8259) (28.6471, -10.823) (28.6413, -10.8202) (28.6357, -10.8175) (28.6301, -10.8148) (28.6247, -10.8122) (28.6194, -10.8097) (28.6142, -10.8073) (28.6091, -10.8049) (28.6042, -10.8026) (28.5994, -10.8004) (28.5947, -10.7983) (28.5902, -10.7962) (28.5858, -10.7942) (28.5816, -10.7923) (28.5775, -10.7905) (28.5736, -10.7888) (28.5698, -10.7871) (28.5661, -10.7855) (28.5626, -10.784) (28.5593, -10.7826) (28.5562, -10.7812) (28.5532, -10.7799) (28.5504, -10.7787) (28.5477, -10.7776) (28.5452, -10.7766) (28.543, -10.7757) (28.5409, -10.7748) (28.5389, -10.774) (28.5372, -10.7733) (28.5357, -10.7727) (28.5344, -10.7722) (28.5336, -10.7719) (28.533, -10.7717) (28.5327, -10.7715) (28.5325, -10.7715) knots -1 -1 -1 -1 -1 -1 -0.99583333 -0.99166667 -0.9875 -0.98333333 -0.97916667 -0.975 -0.97083333 -0.96666667 -0.9625 -0.95833333 -0.95416667 -0.95 -0.94583333 -0.94166667 -0.9375 -0.93333333 -0.92916667 -0.925 -0.92083333 -0.91666667 -0.9125 -0.90833333 -0.90416667 -0.9 -0.89583333 -0.89166667 -0.8875 -0.88333333 -0.87916667 -0.875 -0.87083333 -0.86666667 -0.8625 -0.85833333 -0.85416667 -0.85 -0.84583333 -0.84166667 -0.8375 -0.83333333 -0.82916667 -0.825 -0.82083333 -0.81666667 -0.8125 -0.80833333 -0.80416667 -0.8 -0.79583333 -0.79166667 -0.7875 -0.78333333 -0.77916667 -0.775 -0.77083333 -0.76666667 -0.7625 -0.75833333 -0.75416667 -0.75 -0.74583333 -0.74166667 -0.7375 -0.73333333 -0.72916667 -0.725 -0.72083333 -0.71666667 -0.7125 -0.70833333 -0.70416667 -0.7 -0.69583333 -0.69166667 -0.6875 -0.68333333 -0.67916667 -0.675 -0.67083333 -0.66666667 -0.6625 -0.65833333 -0.65416667 -0.65 -0.64583333 -0.64166667 -0.6375 -0.63333333 -0.62916667 -0.625 -0.62083333 -0.61666667 -0.6125 -0.60833333 -0.60416667 -0.6 -0.59583333 -0.59166667 -0.5875 -0.58333333 -0.57916667 -0.575 -0.57083333 -0.56666667 -0.5625 -0.55833333 -0.55416667 -0.55 -0.54583333 -0.54166667 -0.5375 -0.53333333 -0.52916667 -0.525 -0.52083333 -0.51666667 -0.5125 -0.50833333 -0.50416667 -0.5 -0.49583333 -0.49166667 -0.4875 -0.48333333 -0.47916667 -0.475 -0.47083333 -0.46666667 -0.4625 -0.45833333 -0.45416667 -0.45 -0.44583333 -0.44166667 -0.4375 -0.43333333 -0.42916667 -0.425 -0.42083333 -0.41666667 -0.4125 -0.40833333 -0.40416667 -0.4 -0.39583333 -0.39166667 -0.3875 -0.38333333 -0.37916667 -0.375 -0.37083333 -0.36666667 -0.3625 -0.35833333 -0.35416667 -0.35 -0.34583333 -0.34166667 -0.3375 -0.33333333 -0.32916667 -0.325 -0.32083333 -0.31666667 -0.3125 -0.30833333 -0.30416667 -0.3 -0.29583333 -0.29166667 -0.2875 -0.28333333 -0.27916667 -0.275 -0.27083333 -0.26666667 -0.2625 -0.25833333 -0.25416667 -0.25 -0.24583333 -0.24166667 -0.2375 -0.23333333 -0.22916667 -0.225 -0.22083333 -0.21666667 -0.2125 -0.20833333 -0.20416667 -0.2 -0.19583333 -0.19166667 -0.1875 -0.18333333 -0.17916667 -0.175 -0.17083333 -0.16666667 -0.1625 -0.15833333 -0.15416667 -0.15 -0.14583333 -0.14166667 -0.1375 -0.13333333 -0.12916667 -0.125 -0.12083333 -0.11666667 -0.1125 -0.10833333 -0.10416667 -0.1 -0.09583333 -0.09166667 -0.0875 -0.08333333 -0.07916667 -0.075 -0.07083333 -0.06666667 -0.0625 -0.05833333 -0.05416667 -0.05 -0.04583333 -0.04166667 -0.0375 -0.03333333 -0.02916667 -0.025 -0.02083333 -0.01666667 -0.0125 -0.00833333 -0.00416667 0 0 0 0 0 0
  line L54 (28.5325, -10.7715) -> (28.5312, -10.771)
  line L55 (28.5312, -10.771) -> (27.0141, -10.1982)
  arc A28 (27.0141, -10.1982) -> (27.8492, -7.6279) centre (0, 0) ccw
  line L56 (27.8492, -7.6279) -> (29.4133, -8.0563)
  line L57 (29.4133, -8.0563) -> (29.4146, -8.0567)
  spline S28 degree 5 poles (29.4146, -8.0567) (29.4148, -8.0567) (29.4151, -8.0568) (29.4157, -8.057) (29.4166, -8.0572) (29.4179, -8.0575) (29.4195, -8.0579) (29.4213, -8.0584) (29.4233, -8.0589) (29.4255, -8.0594) (29.4279, -8.06) (29.4305, -8.0606) (29.4333, -8.0613) (29.4363, -8.062) (29.4395, -8.0627) (29.4428, -8.0635) (29.4463, -8.0643) (29.45, -8.0651) (29.4539, -8.066) (29.458, -8.0668) (29.4622, -8.0677) (29.4666, -8.0687) (29.4711, -8.0696) (29.4758, -8.0706) (29.4807, -8.0716) (29.4857, -8.0726) (29.4909, -8.0736) (29.4962, -8.0747) (29.5017, -8.0757) (29.5073, -8.0768) (29.5131, -8.0779) (29.519, -8.079) (29.5251, -8.0801) (29.5313, -8.0812) (29.5376, -8.0824) (29.5441, -8.0835) (29.5507, -8.0847) (29.5574, -8.0858) (29.5643, -8.087) (29.5713, -8.0882) (29.5784, -8.0893) (29.5857, -8.0905) (29.5931, -8.0917) (29.6006, -8.0929) (29.6082, -8.0941) (29.616, -8.0953) (29.6238, -8.0965) (29.6318, -8.0976) (29.6399, -8.0988) (29.6482, -8.1) (29.6565, -8.1012) (29.665, -8.1024) (29.6736, -8.1036) (29.6822, -8.1047) (29.691, -8.1059) (29.6999, -8.1071) (29.709, -8.1082) (29.7181, -8.1094) (29.7273, -8.1105) (29.7367, -8.1117) (29.7461, -8.1128) (29.7556, -8.1139) (29.7653, -8.1151) (29.775, -8.1162) (29.7849, -8.1173) (29.7949, -8.1184) (29.8049, -8.1194) (29.8151, -8.1205) (29.8253, -8.1216) (29.8357, -8.1226) (29.8461, -8.1237) (29.8567, -8.1247) (29.8673, -8.1257) (29.878, -8.1267) (29.8888, -8.1277) (29.8998, -8.1286) (29.9108, -8.1296) (29.9219, -8.1305) (29.9331, -8.1315) (29.9443, -8.1324) (29.9557, -8.1333) (29.9672, -8.1342) (29.9787, -8.135) (29.9904, -8.1359) (30.0021, -8.1367) (30.0139, -8.1375) (30.0258, -8.1383) (30.0378, -8.1391) (30.0498, -8.1399) (30.062, -8.1406) (30.0742, -8.1413) (30.0865, -8.142) (30.0989, -8.1427) (30.1114, -8.1434) (30.1239, -8.144) (30.1365, -8.1446) (30.1493, -8.1453) (30.162, -8.1458) (30.1749, -8.1464) (30.1879, -8.1469) (30.2009, -8.1475) (30.214, -8.148) (30.2272, -8.1485) (30.2404, -8.1489) (30.2537, -8.1493) (30.2671, -8.1498) (30.2806, -8.1501) (30.2942, -8.1505) (30.3078, -8.1509) (30.3215, -8.1512) (30.3353, -8.1515) (30.3491, -8.1517) (30.363, -8.152) (30.377, -8.1522) (30.3911, -8.1524) (30.4052, -8.1526) (30.4194, -8.1527) (30.4337, -8.1529) (30.448, -8.153) (30.4624, -8.153) (30.4769, -8.1531) (30.4914, -8.1531) (30.506, -8.1531) (30.5207, -8.1531) (30.5354, -8.153) (30.5502, -8.1529) (30.5651, -8.1528) (30.58, -8.1527) (30.595, -8.1525) (30.6101, -8.1523) (30.6252, -8.1521) (30.6404, -8.1519) (30.6557, -8.1516) (30.671, -8.1513) (30.6864, -8.151) (30.7018, -8.1506) (30.7173, -8.1502) (30.7329, -8.1498) (30.7485, -8.1494) (30.7642, -8.1489) (30.78, -8.1484) (30.7958, -8.1479) (30.8116, -8.1473) (30.8276, -8.1467) (30.8436, -8.1461) (30.8596, -8.1454) (30.8757, -8.1447) (30.8919, -8.144) (30.9081, -8.1433) (30.9244, -8.1425) (30.9407, -8.1417) (30.9571, -8.1409) (30.9736, -8.14) (30.9901, -8.1391) (31.0066, -8.1382) (31.0233, -8.1373) (31.0399, -8.1363) (31.0567, -8.1353) (31.0734, -8.1342) (31.0903, -8.1331) (31.1072, -8.132) (31.1241, -8.1309) (31.1411, -8.1297) (31.1582, -8.1285) (31.1753, -8.1272) (31.1924, -8.126) (31.2097, -8.1247) (31.2269, -8.1233) (31.2442, -8.1219) (31.2616, -8.1205) (31.279, -8.1191) (31.2965, -8.1176) (31.314, -8.1161) (31.3316, -8.1146) (31.3492, -8.113) (31.3669, -8.1114) (31.3846, -8.1098) (31.4024, -8.1081) (31.4202, -8.1064) (31.4381, -8.1047) (31.456, -8.1029) (31.4739, -8.1011) (31.492, -8.0993) (31.51, -8.0974) (31.5281, -8.0955) (31.5463, -8.0935) (31.5645, -8.0915) (31.5828, -8.0895) (31.601, -8.0875) (31.6194, -8.0854) (31.6378, -8.0833) (31.6562, -8.0811) (31.6747, -8.0789) (31.6932, -8.0767) (31.7118, -8.0745) (31.7304, -8.0722) (31.7491, -8.0698) (31.7678, -8.0675) (31.7866, -8.0651) (31.8054, -8.0626) (31.8242, -8.0602) (31.8431, -8.0577) (31.862, -8.0551) (31.881, -8.0525) (31.9, -8.0499) (31.9191, -8.0473) (31.9382, -8.0446) (31.9573, -8.0419) (31.9765, -8.0391) (31.9957, -8.0363) (32.015, -8.0335) (32.0343, -8.0306) (32.0537, -8.0277) (32.0731, -8.0248) (32.0925, -8.0218) (32.112, -8.0188) (32.1315, -8.0157) (32.151, -8.0126) (32.1706, -8.0095) (32.1903, -8.0063) (32.2099, -8.0031) (32.2297, -7.9999) (32.2494, -7.9966) (32.2692, -7.9933) (32.289, -7.99) (32.3089, -7.9866) (32.3288, -7.9831) (32.3488, -7.9797) (32.3688, -7.9762) (32.3888, -7.9726) (32.4088, -7.9691) (32.4289, -7.9655) (32.4491, -7.9618) (32.4693, -7.9581) (32.4895, -7.9544) (32.5097, -7.9506) (32.53, -7.9468) (32.5503, -7.943) (32.5707, -7.9391) (32.5911, -7.9352) (32.6115, -7.9312) (32.6279, -7.928) (32.6402, -7.9256) (32.6484, -7.924) (32.6525, -7.9232) knots 0 0 0 0 0 0 0.00416667 0.00833333 0.0125 0.01666667 0.02083333 0.025 0.02916667 0.03333333 0.0375 0.04166667 0.04583333 0.05 0.05416667 0.05833333 0.0625 0.06666667 0.07083333 0.075 0.07916667 0.08333333 0.0875 0.09166667 0.09583333 0.1 0.10416667 0.10833333 0.1125 0.11666667 0.12083333 0.125 0.12916667 0.13333333 0.1375 0.14166667 0.14583333 0.15 0.15416667 0.15833333 0.1625 0.16666667 0.17083333 0.175 0.17916667 0.18333333 0.1875 0.19166667 0.19583333 0.2 0.20416667 0.20833333 0.2125 0.21666667 0.22083333 0.225 0.22916667 0.23333333 0.2375 0.24166667 0.24583333 0.25 0.25416667 0.25833333 0.2625 0.26666667 0.27083333 0.275 0.27916667 0.28333333 0.2875 0.29166667 0.29583333 0.3 0.30416667 0.30833333 0.3125 0.31666667 0.32083333 0.325 0.32916667 0.33333333 0.3375 0.34166667 0.34583333 0.35 0.35416667 0.35833333 0.3625 0.36666667 0.37083333 0.375 0.37916667 0.38333333 0.3875 0.39166667 0.39583333 0.4 0.40416667 0.40833333 0.4125 0.41666667 0.42083333 0.425 0.42916667 0.43333333 0.4375 0.44166667 0.44583333 0.45 0.45416667 0.45833333 0.4625 0.46666667 0.47083333 0.475 0.47916667 0.48333333 0.4875 0.49166667 0.49583333 0.5 0.50416667 0.50833333 0.5125 0.51666667 0.52083333 0.525 0.52916667 0.53333333 0.5375 0.54166667 0.54583333 0.55 0.55416667 0.55833333 0.5625 0.56666667 0.57083333 0.575 0.57916667 0.58333333 0.5875 0.59166667 0.59583333 0.6 0.60416667 0.60833333 0.6125 0.61666667 0.62083333 0.625 0.62916667 0.63333333 0.6375 0.64166667 0.64583333 0.65 0.65416667 0.65833333 0.6625 0.66666667 0.67083333 0.675 0.67916667 0.68333333 0.6875 0.69166667 0.69583333 0.7 0.70416667 0.70833333 0.7125 0.71666667 0.72083333 0.725 0.72916667 0.73333333 0.7375 0.74166667 0.74583333 0.75 0.75416667 0.75833333 0.7625 0.76666667 0.77083333 0.775 0.77916667 0.78333333 0.7875 0.79166667 0.79583333 0.8 0.80416667 0.80833333 0.8125 0.81666667 0.82083333 0.825 0.82916667 0.83333333 0.8375 0.84166667 0.84583333 0.85 0.85416667 0.85833333 0.8625 0.86666667 0.87083333 0.875 0.87916667 0.88333333 0.8875 0.89166667 0.89583333 0.9 0.90416667 0.90833333 0.9125 0.91666667 0.92083333 0.925 0.92916667 0.93333333 0.9375 0.94166667 0.94583333 0.95 0.95416667 0.95833333 0.9625 0.96666667 0.97083333 0.975 0.97916667 0.98333333 0.9875 0.99166667 0.99583333 1 1 1 1 1 1
  arc A29 (32.6525, -7.9232) -> (33.0522, -6.0428) centre (0, 0) ccw